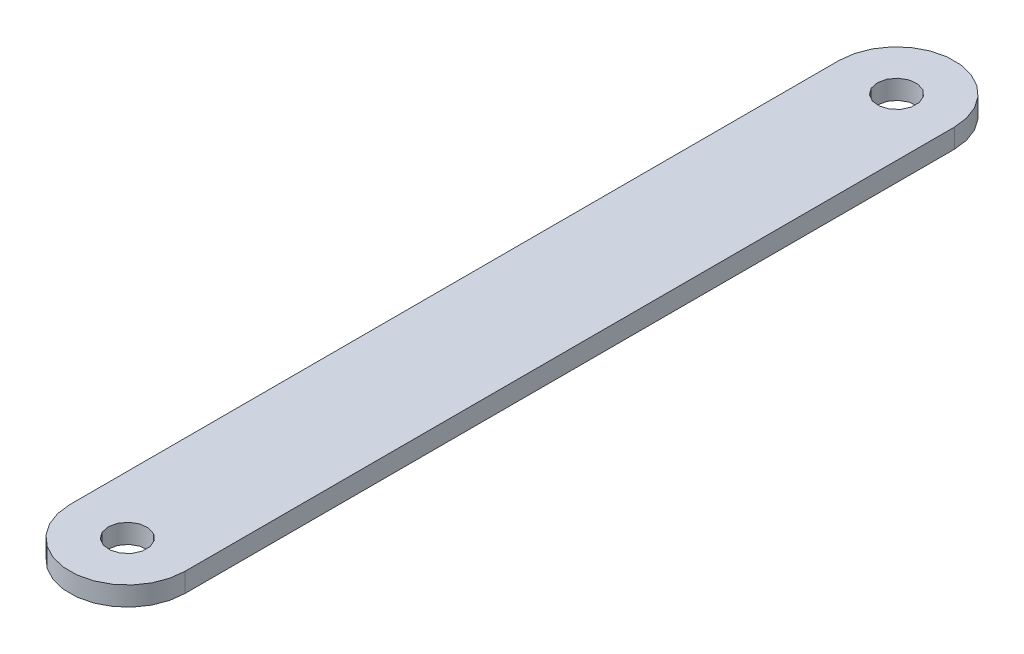
# Autodesk Inventor part: 2AM-17-P-5204 - links
Saved by Autodesk Inventor 2017 (Build 210142000, 142)
## iProperties
Created: 2017-09-30
Part Number: 2AM-17-P-5204 - links
Material: Aluminum 6061
Document SubType Name: Modeling
Designer: Gus
Density: 2.7 g/cm^3
Appearance: Aluminum - Flat
Mass: 22.6403 g
Surface Area: 64.0521 cm^2
Volume: 8.38528 cm^3
Author: Gus
Autodesk Inventor part; units mm, degrees
ref_plane "YZ Plane" through (0, 0, 0) normal (1, 0, 0) x (0, 1, 0)
ref_plane "XZ Plane" through (0, 0, 0) normal (0, 1, 0) x (-1, 0, 0)
ref_plane "XY Plane" through (0, 0, 0) normal (0, 0, 1) x (1, 0, 0)
sketch "Sketch1" plane through (0, 0, 0) normal (0, 1, 0) x (-1, 0, 0)
  line L0 (0, 0) -> (0, -127) construction
  line L1 (-9.525, 0) -> (-9.525, -127)
  line L2 (9.525, -127) -> (9.525, 0)
  arc A0 (9.525, 0) -> (-9.525, 0) centre (0, 0) ccw
  arc A1 (-9.525, -127) -> (9.525, -127) centre (0, -127) ccw
  circle A2 centre (0, 0) radius 3.175
  circle A3 centre (0, -127) radius 3.175
  point P0 (0, -63.5)
  dimension "d0" = 127
  dimension "d1" = 19.05
  dimension "d2" = 6.35
  dimension "d3" = 6.35
  constraints: 8 end point, 4 centre point, 4 point on circle, 4 tangent, 2 coincident, 1 midpoint, 1 parallel, 1 vertical
  measures "d0" distance of L0.start L0.end
  measures "d1" diameter of A1
  measures "d2" diameter of A2
  measures "d3" diameter of A3
extrude "Extrusion1" add sketch "Sketch1" along normal blind 3.175
body "Solid1"
